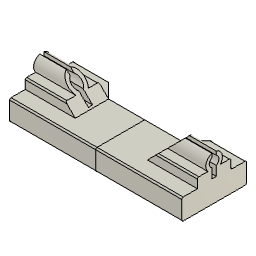
Refelctance array mount for XRP (Autodesk Fusion 360 design; units mm, degrees)
Autodesk Fusion 360 part; units mm, degrees
sketch "Sketch2" plane through (0, 0, 0) normal (1, 0, 0) x (0, 1, 0)
  line L0 (0, 0) -> (-11.65, 0)
  line L1 (-11.65, 0) -> (-11.65, -7.5)
  line L2 (-11.65, -7.5) -> (-10.25, -7.5)
  line L3 (-9.25, -6.5) -> (-10.05, -6.5)
  line L4 (-10.05, -6.5) -> (-10.05, -4.8)
  line L5 (-10.05, -4.8) -> (-8.45, -4.8)
  line L6 (-8.45, -4.8) -> (-8.45, -3.2)
  line L7 (-8.45, -3.2) -> (-10.05, -3.2)
  line L8 (-10.05, -3.2) -> (-10.05, -1.6)
  line L9 (-10.05, -1.6) -> (0, -1.6)
  line L10 (0, -1.6) -> (0, 0)
  line L11 (-9.25, -6.5) -> (-9.25, -6.7)
  line L12 (-9.25, -6.7) -> (-10.25, -7.5)
  circle A0 centre (0, 5.5) radius 3
  line L13 (9.25, -6.5) -> (10.05, -6.5)
  line L14 (10.05, -1.6) -> (0, -1.6)
  line L15 (10.05, -3.2) -> (10.05, -1.6)
  line L16 (0, -1.6) -> (0, 0)
  line L17 (8.45, -3.2) -> (10.05, -3.2)
  line L18 (9.25, -6.5) -> (9.25, -6.7)
  line L19 (0, 0) -> (11.65, 0)
  line L20 (10.05, -4.8) -> (8.45, -4.8)
  line L21 (9.25, -6.7) -> (10.25, -7.5)
  line L22 (8.45, -4.8) -> (8.45, -3.2)
  line L23 (10.05, -6.5) -> (10.05, -4.8)
  line L24 (11.65, -7.5) -> (10.25, -7.5)
  line L25 (11.65, 0) -> (11.65, -7.5)
  circle A1 centre (0, 5.5) radius 1.75
  line L26 (-6, 3.5) -> (6, 3.5)
  line L27 (6, 3.5) -> (6, 0)
  line L28 (6, 0) -> (-6, 0)
  line L29 (-6, 0) -> (-6, 3.5)
  line L30 (-0.75, 9.5) -> (0.75, 9.5)
  line L31 (0.75, 9.5) -> (0.75, 0.5)
  line L32 (0.75, 0.5) -> (-0.75, 0.5)
  line L33 (-0.75, 0.5) -> (-0.75, 9.5)
  line L34 (-11.65, -7.5) -> (11.65, -7.5)
  point P0 (0, 0.5)
  dimension "d3" = 1.6
  dimension "d5" = 0.2
  dimension "d6" = 1.4
  dimension "d7" = 1
  dimension "d8" = 0.8
  dimension "d9" = 7.5
  dimension "d10" = 10.05
  dimension "d11" = 1.6
  dimension "d12" = 1.6
  dimension "d13" = 1.6
  dimension "d14" = 1.7
  dimension "d15" = 0.8
  dimension "d16" = 6
  dimension "d17" = 5.5
  dimension "d18" = 3.5
  dimension "d19" = 2
  dimension "d20" = 12
  dimension "d21" = 5
  dimension "d22" = 1.5
  dimension "d23" = 9
  constraint coincident L0.start L10.end
  constraint horizontal L0
  constraint perpendicular L0 L1
  constraint perpendicular L1 L2
  constraint parallel L2 L3
  constraint perpendicular L3 L4
  constraint perpendicular L4 L5
  constraint perpendicular L3 L6
  constraint perpendicular L4 L7
  constraint perpendicular L7 L8
  constraint perpendicular L4 L9
  constraint perpendicular L0 L10
  constraint perpendicular L3 L11
  constraint collinear L4 L8
  constraint symmetric L0.start L10 L16.end
  constraint symmetric L0.end L10 L19.end
  constraint symmetric L1.end L10 L24.start
  constraint symmetric L2.end L10 L21.end
  constraint symmetric L3.start L10 L13.start
  constraint symmetric L3.end L10 L13.end
  constraint symmetric L4.end L10 L20.start
  constraint symmetric L5.end L10 L20.end
  constraint symmetric L6.end L10 L17.start
  constraint symmetric L7.end L10 L15.start
  constraint symmetric L8.end L10 L14.start
  constraint symmetric L9.end L10 L14.end
  constraint symmetric L10 L11.end L18.end
  constraint vertical A0.centre L0.start
  constraint concentric A0 A1
  constraint horizontal L26
  constraint vertical L27
  constraint horizontal L28
  constraint vertical L29
  constraint coincident L19 L27.end
  constraint midpoint L0.start L28
  constraint horizontal L30
  constraint vertical L31
  constraint horizontal L32
  constraint vertical L33
  constraint midpoint L32 P0
  constraint vertical A0.centre P0
  measures "d3" distance of L9.end L0.start
  measures "d5" distance of L3.start L11.end
  measures "d6" distance of L1.end L2.end
  measures "d7" horizontal distance of L2.end L11.end
  measures "d8" vertical distance of L2.end L11.end
  measures "d9" distance of L0.end L1.end
  measures "d10" distance of L8.end L9.end
  measures "d11" distance of L7.end L8.end
  measures "d12" distance of L6.end L7.end
  measures "d13" distance of L5.end L6.end
  measures "d14" distance of L3.end L4.end
  measures "d15" distance of L3.start L3.end
  measures "d16" diameter of A0
  measures "d17" vertical distance of L0.start A0.centre
  measures "d18" diameter of A1
  measures "d19" vertical distance of A0.centre L26.end
  measures "d20" distance of L26.start L26.end
  measures "d21" vertical distance of A0.centre L32.end
  measures "d22" distance of L30.start L30.end
  measures "d23" distance of L30.end L31.end
extrude "Extrude1" add sketch "Sketch2" along normal blind 31 contours L0 L1 L2 L3 L4 L5 L6 L7 L8 L9 L10 L11 L12 L16 L28 L34 | L10 L13 L14 L15 L16 L17 L18 L19 L20 L21 L22 L23 L24 L25 L28 L34 | L0 A0 L19 L26 L27 L28 L29 L31 L32 L33 | A0 L26 L33 | A0 A1 L26 L33 | A0 A1 L26 L31 | A0 L26 L31 makes body 1
extrude "Extrude4" add sketch "Sketch2" along normal blind 1 from surface at 30 contours L0 L1 L2 L3 L4 L5 L6 L7 L8 L9 L10 L11 L12 L16 L28 L34 | L10 L13 L14 L15 L16 L17 L18 L19 L20 L21 L22 L23 L24 L25 L28 L34 | L3 L4 L5 L6 L7 L8 L9 L11 L12 L13 L14 L15 L17 L18 L20 L21 L22 L23 L34 bodies 1
sketch "Sketch3" plane through (0, 0, 0) normal (0, 1, 0) x (1, 0, 0)
  line L0 (0, 0) -> (13, 0)
  line L1 (13, 0) -> (22, -9)
  line L2 (22, -9) -> (0, -9)
  line L3 (0, -9) -> (0, 0)
  point P0 (0, -9)
  dimension "d28" = 135
  dimension "d37" = 9
  dimension "d38" = 22
  constraint coincident L0.start L3.end
  constraint horizontal L0
  constraint vertical L0.start L2.end
  constraint coincident P0 L2.end
  constraint horizontal L2
  measures "d28" angle of L0 L1
  measures "d37" distance of P0 L0.start
  measures "d38" distance of L1.end P0
extrude "Extrude2" cut sketch "Sketch3" along normal through all and the other way through all bodies 1
sketch "Sketch4" plane through (0, 0, 0) normal (0, 0, 1) x (-1, 0, 0)
  line L0 (0, 11.65) -> (-31, 11.65)
  line L1 (-31, 11.65) -> (-31, 6)
  line L2 (-31, 6) -> (-13, 6)
  line L3 (-13, 6) -> (-13, -6)
  line L4 (-13, -6) -> (-31, -6)
  line L5 (-31, -6) -> (-31, -11.65)
  line L6 (-31, -11.65) -> (0, -11.65)
  line L7 (0, -11.65) -> (0, 11.65)
  line L8 (-13, -6) -> (0, -6)
  line L9 (-13, -6) -> (-20, -13)
  line L10 (-13, -6) -> (-10.1299, -6) construction
  line L11 (-20, -13) -> (0, -13)
  line L12 (0, -13) -> (0, -6)
  arc A0 (-17, -10) -> (-18.6, -8.4) centre (-18.6, -10) ccw
  line L13 (-18.6, -10) -> (-17, -10) construction
  line L14 (-18.6, -10) -> (-18.6, -8.4) construction
  line L15 (-18.6, -8.4) -> (-18.6, -6)
  line L16 (-13, -6) -> (-18.6, -6)
  point P0 (-17, -10)
  dimension "d46" = 13
  dimension "d47" = 6
  dimension "d48" = 135
  dimension "d49" = 7
  dimension "d50" = 4
  dimension "d51" = 90
  dimension "d52" = 1.6
  constraint coincident L3.end L4.start
  constraint coincident L7 L8.end
  constraint perpendicular L7 L8
  constraint horizontal L10
  constraint perpendicular L7 L11
  constraint perpendicular L8 L12
  constraint coincident L9 P0
  constraint coincident P0 A0.start
  constraint horizontal P0 A0.centre
  constraint coincident L4 L15.end
  constraint perpendicular L4 L15
  measures "d46" distance of L3.end L8.end
  measures "d47" vertical distance of L3.end origin
  measures "d48" angle of L9 L10
  measures "d49" distance of L8.end L11.end
  measures "d50" vertical distance of L8.end P0
  measures "d51" angle of L13 L14
  measures "d52" distance of A0.centre P0
extrude "Extrude3" cut sketch "Sketch4" against normal blind 25 contours L6 L7 L8 L9 L12 bodies 1
extrude "Extrude5" cut sketch "Sketch4" against normal blind 7 from surface at -2 contours L4 L9 A0 L15 L16 bodies 1
fillet "Fillet1" radius 0.5 7 edges at (15.5, -11.65, 0) (23.75, -6, 3.5) (15.5, -11.65, -7.5) (23.75, 6, 3.5) (24.825, 11.65, 0) (15.5, 6, 0) (24.825, 11.65, -7.5) on bodies 1
mirror "Mirror1" about plane through (0, 0, 0) normal (1, 0, 0) of bodies 1 makes body 2
